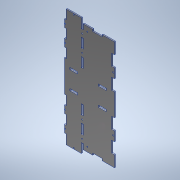
# Autodesk Inventor part: AdaptiveTopPlate03
Saved by Autodesk Inventor 2022 (Build 260153000, 153)
## iProperties
Created: 2021-03-30
Part Number: AdaptiveTopPlate03
Material: Aluminum 6061
Document SubType Name: Modeling
Designer: Esketitttttt
Density: 2.7 g/cm^3
Appearance: Aluminum - Flat
Mass: 5081.03 g
Surface Area: 5064.22 cm^2
Volume: 1881.86 cm^3
Author: Esketitttttt
Autodesk Inventor part; units mm, degrees
ref_plane "YZ Plane" through (0, 0, 0) normal (1, 0, 0) x (0, 1, 0)
ref_plane "XZ Plane" through (0, 0, 0) normal (0, 1, 0) x (-1, 0, 0)
ref_plane "Work Plane1" through (0, 0, 0) normal (0, 0, 1) x (1, 0, 0)
sketch "Sketch1" plane through (0, 0, 0) normal (0, 0, 1) x (1, 0, 0)
  line L0 (0, 30.1625) -> (-12.7, 30.1625) projected
  line L1 (-12.7, -33.3375) -> (-12.7, 30.1625) projected
  line L2 (0, -33.3375) -> (-12.7, -33.3375) projected
  line L3 (0, 30.1625) -> (0, -33.3375) projected
  line L4 (-127, -33.3375) -> (-114.3, -33.3375) projected
  line L5 (-114.3, 30.1625) -> (-114.3, -33.3375) projected
  line L6 (-127, 30.1625) -> (-114.3, 30.1625) projected
  line L7 (-127, -33.3375) -> (-127, 30.1625) projected
  line L8 (-127, 80.3275) -> (-114.3, 80.3275) projected
  line L9 (-114.3, 143.8275) -> (-114.3, 80.3275) projected
  line L10 (-127, 143.8275) -> (-114.3, 143.8275) projected
  line L11 (-127, 80.3275) -> (-127, 143.8275) projected
  line L12 (0, 143.8275) -> (-12.7, 143.8275) projected
  line L13 (-12.7, 80.3275) -> (-12.7, 143.8275) projected
  line L14 (0, 80.3275) -> (-12.7, 80.3275) projected
  line L15 (0, 143.8275) -> (0, 80.3275) projected
  line L16 (64.77, -5.08) -> (128.27, -5.08) projected
  line L17 (128.27, -5.08) -> (128.27, 7.62) projected
  line L18 (64.77, 7.62) -> (128.27, 7.62) projected
  line L19 (64.77, -5.08) -> (64.77, 7.62) projected
  line L20 (-127, 193.9925) -> (-114.3, 193.9925) projected
  line L21 (-114.3, 257.4925) -> (-114.3, 193.9925) projected
  line L22 (-127, 257.4925) -> (-114.3, 257.4925) projected
  line L23 (-127, 193.9925) -> (-127, 257.4925) projected
  line L24 (0, 257.4925) -> (-12.7, 257.4925) projected
  line L25 (-12.7, 193.9925) -> (-12.7, 257.4925) projected
  line L26 (0, 193.9925) -> (-12.7, 193.9925) projected
  line L27 (0, 257.4925) -> (0, 193.9925) projected
  line L28 (212.09, 287.655) -> (193.04, 287.655) projected
  line L29 (193.04, 211.455) -> (193.04, 287.655) projected
  line L30 (212.09, 211.455) -> (193.04, 211.455) projected
  line L31 (212.09, 287.655) -> (212.09, 211.455) projected
  line L32 (212.09, 147.32) -> (193.04, 147.32) projected
  line L33 (193.04, 71.12) -> (193.04, 147.32) projected
  line L34 (212.09, 71.12) -> (193.04, 71.12) projected
  line L35 (212.09, 147.32) -> (212.09, 71.12) projected
  line L36 (154.94, 295.5925) -> (154.94, 308.2925) projected
  line L37 (104.14, 308.2925) -> (154.94, 308.2925) projected
  line L38 (104.14, 295.5925) -> (104.14, 308.2925) projected
  line L39 (154.94, 295.5925) -> (104.14, 295.5925) projected
  line L40 (-38.1, 295.5925) -> (-38.1, 308.2925) projected
  line L41 (-88.9, 308.2925) -> (-38.1, 308.2925) projected
  line L42 (-88.9, 295.5925) -> (-88.9, 308.2925) projected
  line L43 (-38.1, 295.5925) -> (-88.9, 295.5925) projected
  line L44 (-38.1, 419.4175) -> (-38.1, 432.1175) projected
  line L45 (-88.9, 432.1175) -> (-38.1, 432.1175) projected
  line L46 (-88.9, 419.4175) -> (-88.9, 432.1175) projected
  line L47 (-38.1, 419.4175) -> (-88.9, 419.4175) projected
  line L48 (154.94, 419.4175) -> (154.94, 432.1175) projected
  line L49 (104.14, 432.1175) -> (154.94, 432.1175) projected
  line L50 (104.14, 419.4175) -> (104.14, 432.1175) projected
  line L51 (154.94, 419.4175) -> (104.14, 419.4175) projected
  line L52 (212.09, 516.255) -> (193.04, 516.255) projected
  line L53 (193.04, 440.055) -> (193.04, 516.255) projected
  line L54 (212.09, 440.055) -> (193.04, 440.055) projected
  line L55 (212.09, 516.255) -> (212.09, 440.055) projected
  line L56 (212.09, 656.59) -> (193.04, 656.59) projected
  line L57 (193.04, 580.39) -> (193.04, 656.59) projected
  line L58 (212.09, 580.39) -> (193.04, 580.39) projected
  line L59 (212.09, 656.59) -> (212.09, 580.39) projected
  line L60 (-127, 470.2175) -> (-114.3, 470.2175) projected
  line L61 (-114.3, 533.7175) -> (-114.3, 470.2175) projected
  line L62 (-127, 533.7175) -> (-114.3, 533.7175) projected
  line L63 (-127, 470.2175) -> (-127, 533.7175) projected
  line L64 (-127, 583.8825) -> (-114.3, 583.8825) projected
  line L65 (-114.3, 647.3825) -> (-114.3, 583.8825) projected
  line L66 (-127, 647.3825) -> (-114.3, 647.3825) projected
  line L67 (-127, 583.8825) -> (-127, 647.3825) projected
  line L68 (-127, 697.5475) -> (-114.3, 697.5475) projected
  line L69 (-114.3, 761.0475) -> (-114.3, 697.5475) projected
  line L70 (-127, 761.0475) -> (-114.3, 761.0475) projected
  line L71 (-127, 697.5475) -> (-127, 761.0475) projected
  line L72 (0, 761.0475) -> (-12.7, 761.0475) projected
  line L73 (-12.7, 697.5475) -> (-12.7, 761.0475) projected
  line L74 (0, 697.5475) -> (-12.7, 697.5475) projected
  line L75 (0, 761.0475) -> (0, 697.5475) projected
  line L76 (0, 647.3825) -> (-12.7, 647.3825) projected
  line L77 (-12.7, 583.8825) -> (-12.7, 647.3825) projected
  line L78 (0, 583.8825) -> (-12.7, 583.8825) projected
  line L79 (0, 647.3825) -> (0, 583.8825) projected
  line L80 (64.77, 720.09) -> (128.27, 720.09) projected
  line L81 (128.27, 720.09) -> (128.27, 732.79) projected
  line L82 (64.77, 732.79) -> (128.27, 732.79) projected
  line L83 (64.77, 720.09) -> (64.77, 732.79) projected
  line L84 (0, 533.7175) -> (-12.7, 533.7175) projected
  line L85 (-12.7, 470.2175) -> (-12.7, 533.7175) projected
  line L86 (0, 470.2175) -> (-12.7, 470.2175) projected
  line L87 (0, 533.7175) -> (0, 470.2175) projected
  circle A0 centre (28.575, 700.7225) radius 3.175
  circle A1 centre (28.575, 26.9875) radius 3.175
  line L88 (212.09, 172.6438) -> (193.04, 172.6438) projected
  line L89 (193.04, 147.32) -> (193.04, 172.6438) projected
  line L90 (212.09, 147.32) -> (193.04, 147.32) projected
  line L91 (212.09, 172.6438) -> (212.09, 147.32) projected
  line L92 (212.09, 211.455) -> (193.04, 211.455) projected
  line L93 (193.04, 186.1312) -> (193.04, 211.455) projected
  line L94 (212.09, 186.1312) -> (193.04, 186.1312) projected
  line L95 (212.09, 211.455) -> (212.09, 186.1312) projected
  line L96 (193.04, 541.5788) -> (212.09, 541.5788) projected
  line L97 (193.04, 516.255) -> (193.04, 541.5788) projected
  line L98 (212.09, 516.255) -> (193.04, 516.255) projected
  line L99 (212.09, 541.5788) -> (212.09, 516.255) projected
  line L100 (-69.85, 741.5742) -> (-69.85, 712.9992) projected
  line L101 (-69.85, 712.9992) -> (-12.7, 712.9992) projected
  line L102 (-12.7, 712.9992) -> (-12.7, 748.3475) projected
  line L103 (-12.7, 741.5742) -> (-69.85, 741.5742) projected
  circle A2 centre (-41.275, 716.9679) radius 2.0193 projected
  circle A3 centre (-41.275, 737.6054) radius 2.0193 projected
  circle A4 centre (-41.275, 727.2867) radius 3.175 projected
  line L104 (-114.3, -33.3375) -> (-114.3, -20.6375) projected
  line L105 (-70.2437, -33.3375) -> (-114.3, -33.3375) projected
  line L106 (-70.2437, -20.6375) -> (-70.2437, -33.3375) projected
  line L107 (-114.3, -20.6375) -> (-70.2437, -20.6375) projected
  line L108 (-56.7563, -20.6375) -> (-56.7563, -33.3375) projected
  line L109 (-12.7, -33.3375) -> (-56.7563, -33.3375) projected
  line L110 (-12.7, -20.6375) -> (-12.7, -33.3375) projected
  line L111 (-56.7563, -20.6375) -> (-12.7, -20.6375) projected
  line L112 (-127, 30.1625) -> (-114.3, 30.1625) projected
  line L113 (-114.3, 48.5013) -> (-114.3, 30.1625) projected
  line L114 (-127, 48.5013) -> (-114.3, 48.5013) projected
  line L115 (-127, 30.1625) -> (-127, 48.5013) projected
  line L116 (-127, 61.9887) -> (-114.3, 61.9887) projected
  line L117 (-114.3, 80.3275) -> (-114.3, 61.9887) projected
  line L118 (-114.3, 80.3275) -> (-127, 80.3275) projected
  line L119 (-127, 61.9887) -> (-127, 80.3275) projected
  line L120 (0, 48.5013) -> (-12.7, 48.5013) projected
  line L121 (-12.7, 30.1625) -> (-12.7, 48.5013) projected
  line L122 (0, 30.1625) -> (-12.7, 30.1625) projected
  line L123 (0, 48.5013) -> (0, 30.1625) projected
  line L124 (0, 80.3275) -> (-12.7, 80.3275) projected
  line L125 (-12.7, 61.9887) -> (-12.7, 80.3275) projected
  line L126 (0, 61.9887) -> (-12.7, 61.9887) projected
  line L127 (0, 80.3275) -> (0, 61.9887) projected
  line L128 (0, 162.1663) -> (-12.7, 162.1663) projected
  line L129 (-12.7, 143.8275) -> (-12.7, 162.1663) projected
  line L130 (0, 143.8275) -> (-12.7, 143.8275) projected
  line L131 (0, 162.1663) -> (0, 143.8275) projected
  line L132 (0, 193.9925) -> (-12.7, 193.9925) projected
  line L133 (-12.7, 175.6537) -> (-12.7, 193.9925) projected
  line L134 (0, 175.6537) -> (-12.7, 175.6537) projected
  line L135 (0, 193.9925) -> (0, 175.6537) projected
  line L136 (-127, 143.8275) -> (-114.3, 143.8275) projected
  line L137 (-114.3, 162.1663) -> (-114.3, 143.8275) projected
  line L138 (-127, 162.1663) -> (-114.3, 162.1663) projected
  line L139 (-127, 143.8275) -> (-127, 162.1663) projected
  line L140 (-127, 175.6537) -> (-114.3, 175.6537) projected
  line L141 (-114.3, 193.9925) -> (-114.3, 175.6537) projected
  line L142 (-127, 193.9925) -> (-114.3, 193.9925) projected
  line L143 (-127, 175.6537) -> (-127, 193.9925) projected
  line L144 (-127, 533.7175) -> (-114.3, 533.7175) projected
  line L145 (-114.3, 552.0563) -> (-114.3, 533.7175) projected
  line L146 (-127, 552.0563) -> (-114.3, 552.0563) projected
  line L147 (-127, 533.7175) -> (-127, 552.0563) projected
  line L148 (-127, 565.5437) -> (-114.3, 565.5437) projected
  line L149 (-114.3, 583.8825) -> (-114.3, 565.5437) projected
  line L150 (-127, 583.8825) -> (-114.3, 583.8825) projected
  line L151 (-127, 565.5437) -> (-127, 583.8825) projected
  line L152 (0, 552.0563) -> (-12.7, 552.0563) projected
  line L153 (-12.7, 533.7175) -> (-12.7, 552.0563) projected
  line L154 (0, 533.7175) -> (-12.7, 533.7175) projected
  line L155 (0, 552.0563) -> (0, 533.7175) projected
  line L156 (0, 583.8825) -> (-12.7, 583.8825) projected
  line L157 (-12.7, 565.5437) -> (-12.7, 583.8825) projected
  line L158 (0, 565.5437) -> (-12.7, 565.5437) projected
  line L159 (0, 583.8825) -> (0, 565.5437) projected
  line L160 (-127, 647.3825) -> (-114.3, 647.3825) projected
  line L161 (-114.3, 665.7213) -> (-114.3, 647.3825) projected
  line L162 (-127, 665.7213) -> (-114.3, 665.7213) projected
  line L163 (-127, 647.3825) -> (-127, 665.7213) projected
  line L164 (-127, 679.2087) -> (-114.3, 679.2087) projected
  line L165 (-114.3, 697.5475) -> (-114.3, 679.2087) projected
  line L166 (-127, 697.5475) -> (-114.3, 697.5475) projected
  line L167 (-127, 679.2087) -> (-127, 697.5475) projected
  line L168 (0, 697.5475) -> (-12.7, 697.5475) projected
  line L169 (-12.7, 679.2087) -> (-12.7, 697.5475) projected
  line L170 (0, 679.2087) -> (-12.7, 679.2087) projected
  line L171 (0, 697.5475) -> (0, 679.2087) projected
  line L172 (0, 665.7213) -> (-12.7, 665.7213) projected
  line L173 (-12.7, 647.3825) -> (-12.7, 665.7213) projected
  line L174 (-12.7, 647.3825) -> (0, 647.3825) projected
  line L175 (0, 665.7213) -> (0, 647.3825) projected
  line L176 (-56.7563, 761.0475) -> (-56.7563, 748.3475) projected
  line L177 (-12.7, 748.3475) -> (-56.7563, 748.3475) projected
  line L178 (-12.7, 761.0475) -> (-12.7, 748.3475) projected
  line L179 (-56.7563, 761.0475) -> (-12.7, 761.0475) projected
  line L180 (-114.3, 748.3475) -> (-114.3, 761.0475) projected
  line L181 (-70.2437, 748.3475) -> (-114.3, 748.3475) projected
  line L182 (-70.2437, 761.0475) -> (-70.2437, 748.3475) projected
  line L183 (-114.3, 761.0475) -> (-70.2437, 761.0475) projected
  line L184 (212.09, 580.39) -> (193.04, 580.39) projected
  line L185 (193.04, 555.0662) -> (193.04, 580.39) projected
  line L186 (212.09, 555.0662) -> (193.04, 555.0662) projected
  line L187 (212.09, 580.39) -> (212.09, 555.0662) projected
  line L188 (212.09, 172.6438) -> (193.04, 186.1312) construction
  line L189 (212.09, 541.5788) -> (193.04, 555.0662) construction
  line L190 (-70.2437, 748.3475) -> (-56.7563, 761.0475) construction
  line L191 (-127, 665.7213) -> (-114.3, 679.2087) construction
  line L192 (-12.7, 665.7213) -> (0, 679.2087) construction
  line L193 (-12.7, 552.0563) -> (0, 565.5437) construction
  line L194 (-127, 552.0563) -> (-114.3, 565.5437) construction
  line L195 (-127, 162.1663) -> (-114.3, 175.6537) construction
  line L196 (-127, 48.5013) -> (-114.3, 61.9887) construction
  line L197 (-12.7, 48.5013) -> (0, 61.9887) construction
  line L198 (-12.7, 162.1663) -> (0, 175.6537) construction
  line L199 (-70.2437, -33.3375) -> (-56.7563, -20.6375) construction
  circle A5 centre (-120.65, 55.245) radius 3.81
  circle A6 centre (-120.65, 168.91) radius 3.81
  circle A7 centre (-6.35, 168.91) radius 3.81
  circle A8 centre (-6.35, 55.245) radius 3.81
  circle A9 centre (-63.5, -26.9875) radius 3.81
  circle A10 centre (202.565, 179.3875) radius 3.81
  circle A11 centre (202.565, 548.3225) radius 3.81
  circle A12 centre (-63.5, 754.6975) radius 3.81
  circle A13 centre (-6.35, 672.465) radius 3.81
  circle A14 centre (-120.65, 672.465) radius 3.81
  circle A15 centre (-120.65, 558.8) radius 3.81
  circle A16 centre (-6.35, 558.8) radius 3.81
  point P0 (0, 0)
  dimension "t" = 7.62
  dimension "d10" = 7.62
  dimension "d11" = 7.62
  dimension "d12" = 7.62
  dimension "d13" = 7.62
  dimension "d14" = 7.62
  dimension "d15" = 7.62
  dimension "d16" = 7.62
  dimension "d17" = 7.62
  dimension "d18" = 7.62
  dimension "d19" = 7.62
  dimension "d20" = 7.62
  constraints: 24 end point, 14 centre point, 12 coincident, 12 midpoint, 8 parallel, 5 other
  measures "t" diameter of A5
  measures "d10" diameter of A6
  measures "d11" diameter of A7
  measures "d12" diameter of A8
  measures "d13" diameter of A9
  measures "d14" diameter of A10
  measures "d15" diameter of A11
  measures "d16" diameter of A12
  measures "d17" diameter of A13
  measures "d18" diameter of A14
  measures "d19" diameter of A15
  measures "d20" diameter of A16
sketch "Sketch2" plane through (-166.37, -390.4192, 0) normal (0, 0, 1) x (0, 1, 0)
  line L0 (357.0817, -39.37) -> (1151.4667, -39.37)
  line L1 (1151.4667, -39.37) -> (1151.4667, -378.46)
  line L2 (1151.4667, -378.46) -> (357.0817, -378.46)
  line L3 (357.0817, -378.46) -> (357.0817, -39.37)
  line L4 (1151.4667, -378.46) -> (1123.2092, -378.46)
  line L5 (1123.2092, -378.46) -> (1123.2092, -160.02)
  line L6 (1123.2092, -160.02) -> (1151.4667, -160.02)
  line L7 (1151.4667, -160.02) -> (1151.4667, -378.46)
  line L8 (357.0817, -378.46) -> (385.3392, -378.46)
  line L9 (385.3392, -378.46) -> (385.3392, -160.02)
  line L10 (385.3392, -160.02) -> (357.0817, -160.02)
  line L11 (357.0817, -160.02) -> (357.0817, -378.46)
  point P0 (357.0817, -160.02)
  point P1 (385.3392, -378.46)
  dimension "d2" = 794.385
  dimension "d3" = 339.09
  dimension "d0" = 120.65
  dimension "d1" = 28.2575
  constraints: 24 end point, 6 parallel, 3 horizontal, 3 perpendicular, 1 coincident, 1 collinear, 1 point on line
  measures "d2" distance of L1.end L2.end
  measures "d3" distance of L0.end L1.end
  measures "d0" distance between parallel lines of L0 L6
  measures "d1" distance of L5.end L6.end
extrude "Extrusion1" add sketch "Sketch2" along normal blind 7.9375 contours L0 L1 L6 L5 L2 L9 L10 L3
extrude "Extrusion2" cut sketch "Sketch1" along normal through all contours L3 L2 L1 L0 | L7 L6 L5 L4 | L11 L10 L9 L8 | L15 L14 L13 L12 | L19 L18 L17 L16 | L23 L22 L21 L20 | L27 L26 L25 L24 | L31 L30 L29 L28 | L35 L34 L33 L32 | L39 L38 L37 L36 | L43 L42 L41 L40 | L47 L46 L45 L44 | L51 L50 L49 L48 | L55 L54 L53 L52 | L59 L58 L57 L56 | L63 L62 L61 L60 | L67 L66 L65 L64 | L71 L70 L69 L68 | L75 L74 L73 L72 | L79 L78 L77 L76 | L83 L82 L81 L80 | L87 L86 L85 L84 | A0 | A1 | A5 | A6 | A7 | A8 | A9 | A10 | A11 | A12 | A13 | A14 | A15 | A16
equation "\"d10\" = t"
equation "\"d11\" = t"
equation "\"d12\" = t"
equation "\"d13\" = t"
equation "\"d14\" = t"
equation "\"d15\" = t"
equation "\"d16\" = t"
equation "\"d17\" = t"
equation "\"d18\" = t"
equation "\"d19\" = t"
equation "\"d20\" = t"
body "Solid1"
